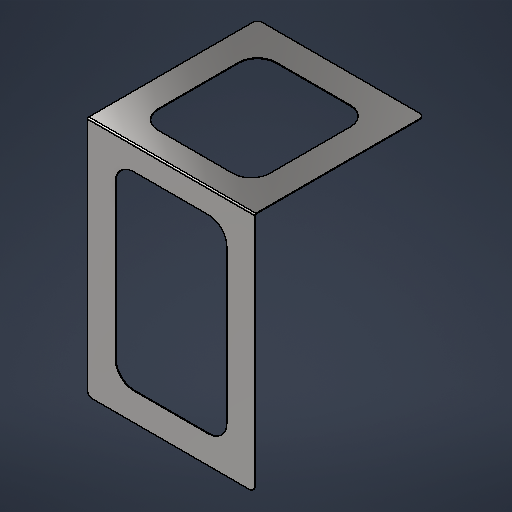
# Autodesk Inventor part: Side Panel
Saved by Autodesk Inventor 2026 (Build 300175050, 175E)
## iProperties
Created: 2025-05-19
Part Number: Side Panel
Material: Steel, Carbon
Document SubType Name: Sheet Metal
Designer: Joshua Eah
Density: 7.85 g/cm^3
Sheet Metal Rule: A36 Steel 20 ga
Appearance: Semi-Polished
Author: Joshua Eah
Autodesk Inventor part; units mm, degrees
ref_plane "YZ Plane" through (0, 0, 0) normal (1, 0, 0) x (0, 1, 0)
ref_plane "XZ Plane" through (0, 0, 0) normal (0, 1, 0) x (-1, 0, 0)
ref_plane "XY Plane" through (0, 0, 0) normal (0, 0, 1) x (1, 0, 0)
sketch "Sketch1" plane through (0, 0, 0) normal (0, 1, 0) x (-1, 0, 0)
  line L0 (0, 0) -> (-230, 0)
  line L1 (-230, 0) -> (-230, -331)
  line L2 (-230, -331) -> (0, -331)
  line L3 (0, -331) -> (0, 0)
  line L4 (-115, -331) -> (-115, 0) construction
  line L5 (-38.1, -299.25) -> (-191.9, -299.25)
  line L6 (-191.9, -299.25) -> (-191.9, -38.1)
  line L7 (-191.9, -38.1) -> (-38.1, -38.1)
  line L8 (-38.1, -38.1) -> (-38.1, -299.25)
  line L9 (-38.1, -299.25) -> (-191.9, -38.1) construction
  line L10 (-191.9, -299.25) -> (-38.1, -38.1) construction
  point P0 (-115, -168.675)
  dimension "d0" = 230
  dimension "d1" = 331
  dimension "d18" = 31.75
  dimension "d20" = 38.1
  dimension "d21" = 38.1
  constraints: 22 end point, 4 midpoint, 4 parallel, 3 perpendicular, 2 horizontal, 1 point on line
  measures "d0" distance of L2.end L1.end
  measures "d1" distance of L1.end L0.end
  measures "d18" distance between parallel lines of L2 L5
  measures "d20" distance between parallel lines of L0 L7
  measures "d21" distance between parallel lines of L3 L8
extrude "Plate1" add sketch "Sketch1" along normal blind 0.9119
sketch "Sketch2" plane through (230, 0.9119, -331.9119) normal (0, 0, 1) x (1, 0, 0)
  line L0 (-230, 0) -> (0, 0)
  line L1 (0, 0) -> (0, -233.9119)
  line L2 (0, -233.9119) -> (-230, -233.9119)
  line L3 (-230, -233.9119) -> (-230, 0)
  constraints: 8 end point
edge flange "Flange1" height 233 angle 90 thickness 0.9119 bend radius 0.9119 thickness toward (0, 0, 1) relief straight relief width 0.9119 relief depth 0.4559 edges at (115, 0, -331) wall of the first edge with corners at (0, 0.9119, -331.9119) (230, 0.9119, -331.9119) (230, -233, -331.9119) (0, -233, -331.9119)
bend "Bend1"
corner "Corner1"
unfold all bends "Unfold1" k factor 0.44 fixed face at (12.7, 0.9119, -122.7294)
sketch "Sketch3" plane through (0, 0.9119, -564.2389) normal (0, 1, 0) x (1, 0, 0)
  line L0 (0, -232.0881) -> (230, -232.0881) projected
  line L1 (230, 0) -> (230, -232.0881) projected
  line L2 (0, 0) -> (230, 0) projected
  line L3 (0, -232.0881) -> (0, 0) projected
  line L4 (38.1, -38.1) -> (191.9, -38.1)
  line L5 (191.9, -38.1) -> (191.9, -200.3381)
  line L6 (191.9, -200.3381) -> (38.1, -200.3381)
  line L7 (38.1, -200.3381) -> (38.1, -38.1)
  point P0 (0, -564.2389)
  dimension "d32" = 38.1
  dimension "d33" = 31.75
  dimension "d34" = 38.1
  dimension "d35" = 38.1
  constraints: 8 end point, 2 parallel, 1 horizontal, 1 perpendicular
  measures "d32" distance between parallel lines of L7 L3
  measures "d33" distance between parallel lines of L0 L6
  measures "d34" distance between parallel lines of L1 L5
  measures "d35" distance between parallel lines of L2 L4
extrude "Extrusion1" cut sketch "Sketch3" against normal through all contours L4 L5 L6 L7
refold all bends "Refold1"
fillet "Corner Round3" radius 6.35 4 edges at (0, 0.4559, 0) (230, 0.4559, 0) (230, -233, -331.4559) (0, -233, -331.4559)
fillet "Corner Round4" radius 25.4 8 edges at (38.1, 0.4559, -299.25) (191.9, 0.4559, -299.25) (191.9, 0.4559, -38.1) (38.1, 0.4559, -38.1) (38.1, -194.9, -331.4559) (191.9, -194.9, -331.4559) (38.1, -32.6619, -331.4559) (191.9, -32.6619, -331.4559)
equation "\"d20\" = d21"
equation "\"d34\" = d32"
equation "\"d35\" = d32"
equation "\"d2\" = Thickness"
equation "\"d22\" = BendReliefWidth"
equation "\"d23\" = BendReliefDepth"
equation "\"d24\" = MinimumRemnant"
equation "\"d25\" = TransitionRadius"
equation "\"d28\" = BendRadius"
equation "\"d29\" = CornerReliefSize"
equation "\"d30\" = GapSize"
equation "\"d31\" = JacobiRadiusSize"
equation "\"BendRadius\" = Thickness"
equation "\"BendReliefWidth\" = Thickness"
equation "\"BendReliefDepth\" = 0.5 * Thickness"
equation "\"CornerReliefSize\" = 4 * Thickness"
equation "\"MinimumRemnant\" = 2 * Thickness"
equation "\"TransitionRadius\" = BendRadius"
equation "\"JacobiRadiusSize\" = BendRadius"
equation "\"GapSize\" = Thickness"
equation "\"Thickness\" = 0.91186"
body "Solid1"
